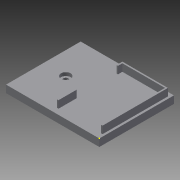
# Autodesk Inventor part: CraneBase
Saved by Autodesk Inventor 2015 (Build 190159000, 159)
## iProperties
Created: 2016-03-18
Part Number: CraneBase
Material: Generic
Document SubType Name: Modeling
Designer: Hatch
Density: 1 g/cm^3
Appearance: Default
Author: Hatch
Autodesk Inventor part; units mm, degrees
ref_plane "YZ Plane" through (0, 0, 0) normal (1, 0, 0) x (0, 1, 0)
ref_plane "XZ Plane" through (0, 0, 0) normal (0, 1, 0) x (-1, 0, 0)
ref_plane "XY Plane" through (0, 0, 0) normal (0, 0, 1) x (1, 0, 0)
sketch "Sketch1" plane through (0, 0, 0) normal (0, 1, 0) x (-1, 0, 0)
  line L0 (0, 0) -> (127, 0)
  line L1 (127, 0) -> (127, -101.6)
  line L2 (127, -101.6) -> (0, -101.6)
  line L3 (0, -101.6) -> (0, 0)
  dimension "d1" = 127
  constraints: 8 end point, 2 parallel, 1 horizontal, 1 perpendicular
  measures "d1" distance of L1.end L2.end
extrude "Extrusion1" add sketch "Sketch1" along normal blind 10
sketch "Sketch2" plane through (0, 10, 0) normal (0, 1, 0) x (1, 0, 0)
  line L0 (0, 0) -> (0, 101.6) projected
  line L1 (-5.9255, 8.3) -> (-61.9255, 8.3)
  line L2 (-61.9255, 8.3) -> (-61.9255, 93.3)
  line L3 (-61.9255, 93.3) -> (-5.9255, 93.3)
  line L4 (-5.9255, 93.3) -> (-5.9255, 8.3)
  line L5 (-5.9255, 8.3) -> (-61.9255, 93.3) construction
  line L6 (-61.9255, 8.3) -> (-5.9255, 93.3) construction
  line L7 (-126.4344, 50.8) -> (-96.4344, 50.8)
  circle A0 centre (-96.4344, 50.8) radius 3.5
  point P0 (-33.9255, 50.8)
  dimension "d5" = 56
  dimension "d6" = 85
  dimension "d7" = 30
  dimension "d8" = 7
  constraints: 14 end point, 2 horizontal, 2 midpoint, 2 parallel, 1 centre point, 1 coincident, 1 perpendicular
  measures "d5" distance of L2.end L3.end
  measures "d6" distance of L1.end L2.end
  measures "d7" distance of L7.start L7.end
  measures "d8" diameter of A0
extrude "Extrusion2" cut sketch "Sketch2" against normal through all contours A0
sketch "Sketch3" plane through (0, 10, 0) normal (0, 1, 0) x (1, 0, 0)
  line L0 (-5.9255, 8.3) -> (-61.9255, 93.3) construction
  line L1 (-61.9255, 8.3) -> (-5.9255, 93.3) construction
  line L2 (-126.4344, 50.8) -> (-96.4344, 50.8)
  circle A0 centre (-96.4344, 50.8) radius 3.5
  line L3 (-4.9255, 7.3) -> (-62.9255, 7.3)
  line L4 (-62.9255, 7.3) -> (-62.9255, 94.3)
  line L5 (-62.9255, 94.3) -> (-4.9255, 94.3)
  line L6 (-4.9255, 94.3) -> (-4.9255, 7.3)
  line L7 (-4.9255, 7.3) -> (-62.9255, 94.3) construction
  line L8 (-62.9255, 7.3) -> (-4.9255, 94.3) construction
  line L9 (-62.9255, 94.3) -> (-62.9255, 84.3)
  line L10 (-62.9255, 94.3) -> (-62.9255, 88.3)
  line L11 (-62.9255, 88.3) -> (-64.9255, 88.3)
  line L12 (-64.9255, 88.3) -> (-64.9255, 96.3)
  line L13 (-64.9255, 96.3) -> (-2.9255, 96.3)
  line L14 (-2.9255, 96.3) -> (-2.9255, 7.3)
  line L15 (-2.9255, 7.3) -> (-4.9255, 7.3)
  line L16 (-4.9255, 94.3) -> (-62.9255, 94.3)
  line L17 (-62.9255, 7.3) -> (-64.9255, 7.3)
  line L18 (-64.9255, 7.3) -> (-64.9255, 32.3)
  line L19 (-64.9255, 32.3) -> (-62.9255, 32.3)
  point P0 (-33.9255, 50.8)
  dimension "d13" = 30
  dimension "d14" = 7
  dimension "d20" = 6
  dimension "d21" = 2
  dimension "d22" = 8
  dimension "d23" = 62
  dimension "d24" = 2
  dimension "d25" = 25
  constraints: 40 end point, 8 perpendicular, 4 midpoint, 3 equal length, 3 horizontal, 3 point on line, 1 centre point, 1 coincident
  measures "d13" distance of L2.start L2.end
  measures "d14" diameter of A0
  measures "d20" distance of L4.end L10.end
  measures "d21" distance of L10.end L11.end
  measures "d22" distance of L11.end L12.end
  measures "d23" distance of L12.end L13.end
  measures "d24" distance of L3.end L17.end
  measures "d25" distance of L17.end L18.end
extrude "Extrusion3" add sketch "Sketch3" along normal blind 10 contours L6 L5 L4 L11 L12 L13 L14 L15 | L17 L18 L19 L4
sketch "Sketch4" plane through (0, 10, 0) normal (0, 1, 0) x (1, 0, 0)
  circle A0 centre (-96.4344, 50.8) radius 3.5 projected
  circle A1 centre (-96.4344, 50.8) radius 6.5
  point P0 (0, 0)
  dimension "d28" = 13
  constraints: 1 centre point, 1 coincident
  measures "d28" diameter of A1
extrude "Extrusion4" cut sketch "Sketch4" against normal blind 4.5
sketch "Sketch5" plane through (0, 10, 0) normal (0, 1, 0) x (1, 0, 0)
  point P0 (0, 0)
body "Solid1"
